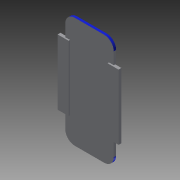
# Autodesk Inventor part: podvozek_priklopny_kryt
Saved by Autodesk Inventor 2015 (Build 190159000, 159)
## iProperties
Created: 2013-08-31
Part Number: podvozek_priklopny_kryt
Material: Generic
Document SubType Name: Modeling
Designer: idle-rug
Density: 1 g/cm^3
Appearance: Default
Author: idle-rug
Autodesk Inventor part; units mm, degrees
ref_plane "YZ Plane" through (0, 0, 0) normal (1, 0, 0) x (0, 1, 0)
ref_plane "XZ Plane" through (0, 0, 0) normal (0, 1, 0) x (-1, 0, 0)
ref_plane "XY Plane" through (0, 0, 0) normal (0, 0, 1) x (1, 0, 0)
sketch "Sketch1" plane through (0, 0, 0) normal (0, 1, 0) x (-1, 0, 0)
  line L0 (50.6, 115.65) -> (-50.6, 115.65)
  line L1 (-50.6, 115.65) -> (-50.6, -115.65)
  line L2 (-50.6, -115.65) -> (50.6, -115.65)
  line L3 (50.6, -115.65) -> (50.6, 115.65)
  line L4 (50.6, 115.65) -> (-50.6, -115.65) construction
  line L5 (-50.6, 115.65) -> (50.6, -115.65) construction
  line L6 (-50.6, -67.1124) -> (-50.6, 70.65)
  line L7 (-50.6, -65.35) -> (-50.6, 70.65)
  line L8 (-50.6, 70.65) -> (-40.6, 70.65)
  line L9 (-40.6, 70.65) -> (-40.6, -65.35)
  line L10 (-40.6, -65.35) -> (-50.6, -65.35)
  line L11 (0, -115.65) -> (0, 115.65)
  line L12 (50.6, -67.1124) -> (50.6, 70.65)
  line L13 (50.6, 70.65) -> (40.6, 70.65)
  line L14 (40.6, 70.65) -> (40.6, -65.35)
  line L15 (40.6, -65.35) -> (50.6, -65.35)
  line L16 (50.6, 70.65) -> (40.6, 70.65)
  line L17 (40.6, 70.65) -> (40.6, -65.35)
  line L18 (40.6, -65.35) -> (50.6, -65.35)
  line L19 (50.6, -65.35) -> (50.6, 70.65)
  line L20 (-40.6, -65.35) -> (-50.6, -65.35)
  line L21 (-50.6, -65.35) -> (-50.6, 70.65)
  line L22 (-50.6, 70.65) -> (-40.6, 70.65)
  line L23 (-40.6, 70.65) -> (-40.6, -65.35)
  point P0 (0, 0)
  dimension "d0" = 231.3
  dimension "d1" = 101.2
  dimension "d14" = 45
  dimension "d18" = 10
  dimension "d19" = 136
  constraints: 48 end point, 6 parallel, 5 perpendicular, 5 symmetric about line, 4 horizontal, 4 midpoint, 2 point on line, 1 collinear
  measures "d0" distance of L0.end L1.end
  measures "d1" distance of L1.end L2.end
  measures "d14" distance of L0.end L6.end
  measures "d18" distance of L6.end L8.end
  measures "d19" distance of L8.end L9.end
extrude "Extrusion1" add sketch "Sketch1" along normal blind 5
fillet "Fillet1" radius 20 4 edges at (-50.6, 2.5, -115.65) (50.6, 2.5, -115.65) (-50.6, 2.5, 115.65) (50.6, 2.5, 115.65)
extrude "Extrusion3" add sketch "Sketch1" against normal blind 3 contours L3 L15 L14 L13 | L8 L9 L10 L1
sketch "Sketch3" plane through (50.6, 0, 95.65) normal (1, 0, 0) x (0, 0, -1)
  line L0 (161, -3) -> (25, -3)
  line L1 (25, -3) -> (25, 3)
  line L2 (25, 3) -> (161, 3)
  line L3 (161, 3) -> (161, -3)
  point P0 (95.65, 0)
  dimension "d22" = 136
  dimension "d23" = 6
  constraints: 8 end point, 2 parallel, 1 horizontal, 1 perpendicular
  measures "d22" distance of L1.end L2.end
  measures "d23" distance of L0.end L1.end
extrude "Extrusion4" add sketch "Sketch3" along normal blind 13
sketch "Sketch4" plane through (-50.6, 0, 95.65) normal (-1, 0, 0) x (0, 0, 1)
  line L0 (-25, -3) -> (-161, -3)
  line L1 (-161, -3) -> (-161, 3)
  line L2 (-161, 3) -> (-25, 3)
  line L3 (-25, 3) -> (-25, -3)
  point P0 (-95.65, 0)
  dimension "d26" = 136
  dimension "d27" = 6
  constraints: 8 end point, 2 parallel, 1 horizontal, 1 perpendicular
  measures "d26" distance of L1.end L2.end
  measures "d27" distance of L0.end L1.end
extrude "Extrusion5" add sketch "Sketch4" along normal blind 13
body "Solid1"
